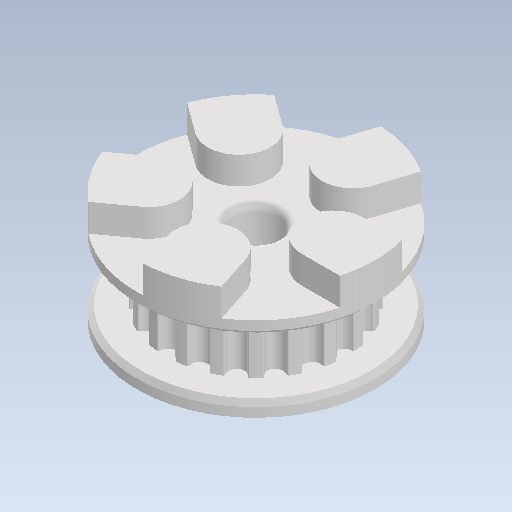
# Autodesk Inventor part: Riemenscheibe HTD_3M
Saved by Autodesk Inventor 2026.4 (Build 304435030, 435C)
## iProperties
Created: 2026-11-19
Part Number: Riemenscheibe HTD_3M
Material: Generisch
Document SubType Name: Modeling
Designer: weira
Density: 1 g/cm^3
Appearance: Vorgabe
Author: weira
Autodesk Inventor part; units mm, degrees
ref_plane "YZ Plane" through (0, 0, 0) normal (1, 0, 0) x (0, 1, 0)
ref_plane "XZ Plane" through (0, 0, 0) normal (0, 1, 0) x (-1, 0, 0)
ref_plane "XY Plane" through (0, 0, 0) normal (0, 0, 1) x (1, 0, 0)
sketch "Skizze1" plane through (0, 0, 0) normal (0, 0, 1) x (1, 0, 0)
  circle A0 centre (0, 0) radius 9.5511 construction
  line L0 (-5.6581, 20.033) -> (2.8903, 20.033)
  line L1 (2.8903, 20.033) -> (2.8903, 11.5277)
  line L2 (2.8903, 11.5277) -> (-5.6581, 11.5277)
  line L3 (-5.6581, 11.5277) -> (-5.6581, 20.033)
  circle A1 centre (0, 0) radius 8.6811 construction
  circle A2 centre (0, 0) radius 9.8211
  arc A3 (0.7095, 9.0476) -> (0.9041, 9.6681) centre (-0.61, 9.8021) ccw
  arc A4 (1.0279, 9.7672) -> (0.9041, 9.6681) centre (1.0264, 9.6422) ccw
  line L4 (0, 8.6811) -> (0, 7.1512) construction
  arc A5 (-0.9041, 9.6681) -> (-0.7095, 9.0476) centre (0.61, 9.8021) ccw
  arc A6 (-0.9041, 9.6681) -> (-1.0279, 9.7672) centre (-1.0264, 9.6422) ccw
  arc A7 (-0.7095, 9.0476) -> (0.7095, 9.0476) centre (0, 9.5511) ccw
  arc A8 (-2.0407, 9.6068) -> (-2.1278, 9.4743) centre (-2.0035, 9.4874) ccw
  arc A9 (-3.8474, 8.9155) -> (-3.9958, 8.9715) centre (-3.9557, 8.8531) ccw
  arc A10 (-2.1211, 8.824) -> (-2.1278, 9.4743) centre (-3.6092, 9.1339) ccw
  arc A11 (-3.8474, 8.9155) -> (-3.4706, 8.3855) centre (-2.4489, 9.5109) ccw
  arc A12 (-3.4706, 8.3855) -> (-2.1211, 8.824) centre (-2.9515, 9.0836) ccw
  arc A13 (-4.9094, 8.506) -> (-4.9513, 8.353) centre (-4.8372, 8.404) ccw
  arc A14 (-6.4142, 7.2902) -> (-6.5726, 7.2976) centre (-6.4979, 7.1974) ccw
  arc A15 (-4.744, 7.7367) -> (-4.9513, 8.353) centre (-6.2551, 7.5715) ccw
  arc A16 (-6.4142, 7.2902) -> (-5.892, 6.9026) centre (-5.2681, 8.2886) ccw
  arc A17 (-5.892, 6.9026) -> (-4.744, 7.7367) centre (-5.614, 7.727) ccw
  arc A18 (-7.2976, 6.5726) -> (-7.2902, 6.4142) centre (-7.1974, 6.4979) ccw
  arc A19 (-8.353, 4.9513) -> (-8.506, 4.9094) centre (-8.404, 4.8372) ccw
  arc A20 (-6.9026, 5.892) -> (-7.2902, 6.4142) centre (-8.2886, 5.2681) ccw
  arc A21 (-8.353, 4.9513) -> (-7.7367, 4.744) centre (-7.5715, 6.2551) ccw
  arc A22 (-7.7367, 4.744) -> (-6.9026, 5.892) centre (-7.727, 5.614) ccw
  arc A23 (-8.9715, 3.9958) -> (-8.9155, 3.8474) centre (-8.8531, 3.9557) ccw
  arc A24 (-9.4743, 2.1278) -> (-9.6068, 2.0407) centre (-9.4874, 2.0035) ccw
  arc A25 (-8.3855, 3.4706) -> (-8.9155, 3.8474) centre (-9.5109, 2.4489) ccw
  arc A26 (-9.4743, 2.1278) -> (-8.824, 2.1211) centre (-9.1339, 3.6092) ccw
  arc A27 (-8.824, 2.1211) -> (-8.3855, 3.4706) centre (-9.0836, 2.9515) ccw
  arc A28 (-9.7672, 1.0279) -> (-9.6681, 0.9041) centre (-9.6422, 1.0264) ccw
  arc A29 (-9.6681, -0.9041) -> (-9.7672, -1.0279) centre (-9.6422, -1.0264) ccw
  arc A30 (-9.0476, 0.7095) -> (-9.6681, 0.9041) centre (-9.8021, -0.61) ccw
  arc A31 (-9.6681, -0.9041) -> (-9.0476, -0.7095) centre (-9.8021, 0.61) ccw
  arc A32 (-9.0476, -0.7095) -> (-9.0476, 0.7095) centre (-9.5511, 0) ccw
  arc A33 (-9.6068, -2.0407) -> (-9.4743, -2.1278) centre (-9.4874, -2.0035) ccw
  arc A34 (-8.9155, -3.8474) -> (-8.9715, -3.9958) centre (-8.8531, -3.9557) ccw
  arc A35 (-8.824, -2.1211) -> (-9.4743, -2.1278) centre (-9.1339, -3.6092) ccw
  arc A36 (-8.9155, -3.8474) -> (-8.3855, -3.4706) centre (-9.5109, -2.4489) ccw
  arc A37 (-8.3855, -3.4706) -> (-8.824, -2.1211) centre (-9.0836, -2.9515) ccw
  arc A38 (-8.506, -4.9094) -> (-8.353, -4.9513) centre (-8.404, -4.8372) ccw
  arc A39 (-7.2902, -6.4142) -> (-7.2976, -6.5726) centre (-7.1974, -6.4979) ccw
  arc A40 (-7.7367, -4.744) -> (-8.353, -4.9513) centre (-7.5715, -6.2551) ccw
  arc A41 (-7.2902, -6.4142) -> (-6.9026, -5.892) centre (-8.2886, -5.2681) ccw
  arc A42 (-6.9026, -5.892) -> (-7.7367, -4.744) centre (-7.727, -5.614) ccw
  arc A43 (-6.5726, -7.2976) -> (-6.4142, -7.2902) centre (-6.4979, -7.1974) ccw
  arc A44 (-4.9513, -8.353) -> (-4.9094, -8.506) centre (-4.8372, -8.404) ccw
  arc A45 (-5.892, -6.9026) -> (-6.4142, -7.2902) centre (-5.2681, -8.2886) ccw
  arc A46 (-4.9513, -8.353) -> (-4.744, -7.7367) centre (-6.2551, -7.5715) ccw
  arc A47 (-4.744, -7.7367) -> (-5.892, -6.9026) centre (-5.614, -7.727) ccw
  arc A48 (-3.9958, -8.9715) -> (-3.8474, -8.9155) centre (-3.9557, -8.8531) ccw
  arc A49 (-2.1278, -9.4743) -> (-2.0407, -9.6068) centre (-2.0035, -9.4874) ccw
  arc A50 (-3.4706, -8.3855) -> (-3.8474, -8.9155) centre (-2.4489, -9.5109) ccw
  arc A51 (-2.1278, -9.4743) -> (-2.1211, -8.824) centre (-3.6092, -9.1339) ccw
  arc A52 (-2.1211, -8.824) -> (-3.4706, -8.3855) centre (-2.9515, -9.0836) ccw
  arc A53 (-1.0279, -9.7672) -> (-0.9041, -9.6681) centre (-1.0264, -9.6422) ccw
  arc A54 (0.9041, -9.6681) -> (1.0279, -9.7672) centre (1.0264, -9.6422) ccw
  arc A55 (-0.7095, -9.0476) -> (-0.9041, -9.6681) centre (0.61, -9.8021) ccw
  arc A56 (0.9041, -9.6681) -> (0.7095, -9.0476) centre (-0.61, -9.8021) ccw
  arc A57 (0.7095, -9.0476) -> (-0.7095, -9.0476) centre (0, -9.5511) ccw
  arc A58 (2.0407, -9.6068) -> (2.1278, -9.4743) centre (2.0035, -9.4874) ccw
  arc A59 (3.8474, -8.9155) -> (3.9958, -8.9715) centre (3.9557, -8.8531) ccw
  arc A60 (2.1211, -8.824) -> (2.1278, -9.4743) centre (3.6092, -9.1339) ccw
  arc A61 (3.8474, -8.9155) -> (3.4706, -8.3855) centre (2.4489, -9.5109) ccw
  arc A62 (3.4706, -8.3855) -> (2.1211, -8.824) centre (2.9515, -9.0836) ccw
  arc A63 (4.9094, -8.506) -> (4.9513, -8.353) centre (4.8372, -8.404) ccw
  arc A64 (6.4142, -7.2902) -> (6.5726, -7.2976) centre (6.4979, -7.1974) ccw
  arc A65 (4.744, -7.7367) -> (4.9513, -8.353) centre (6.2551, -7.5715) ccw
  arc A66 (6.4142, -7.2902) -> (5.892, -6.9026) centre (5.2681, -8.2886) ccw
  arc A67 (5.892, -6.9026) -> (4.744, -7.7367) centre (5.614, -7.727) ccw
  arc A68 (7.2976, -6.5726) -> (7.2902, -6.4142) centre (7.1974, -6.4979) ccw
  arc A69 (8.353, -4.9513) -> (8.506, -4.9094) centre (8.404, -4.8372) ccw
  arc A70 (6.9026, -5.892) -> (7.2902, -6.4142) centre (8.2886, -5.2681) ccw
  arc A71 (8.353, -4.9513) -> (7.7367, -4.744) centre (7.5715, -6.2551) ccw
  arc A72 (7.7367, -4.744) -> (6.9026, -5.892) centre (7.727, -5.614) ccw
  arc A73 (8.9715, -3.9958) -> (8.9155, -3.8474) centre (8.8531, -3.9557) ccw
  arc A74 (9.4743, -2.1278) -> (9.6068, -2.0407) centre (9.4874, -2.0035) ccw
  arc A75 (8.3855, -3.4706) -> (8.9155, -3.8474) centre (9.5109, -2.4489) ccw
  arc A76 (9.4743, -2.1278) -> (8.824, -2.1211) centre (9.1339, -3.6092) ccw
  arc A77 (8.824, -2.1211) -> (8.3855, -3.4706) centre (9.0836, -2.9515) ccw
  arc A78 (9.7672, -1.0279) -> (9.6681, -0.9041) centre (9.6422, -1.0264) ccw
  arc A79 (9.6681, 0.9041) -> (9.7672, 1.0279) centre (9.6422, 1.0264) ccw
  arc A80 (9.0476, -0.7095) -> (9.6681, -0.9041) centre (9.8021, 0.61) ccw
  arc A81 (9.6681, 0.9041) -> (9.0476, 0.7095) centre (9.8021, -0.61) ccw
  arc A82 (9.0476, 0.7095) -> (9.0476, -0.7095) centre (9.5511, 0) ccw
  arc A83 (9.6068, 2.0407) -> (9.4743, 2.1278) centre (9.4874, 2.0035) ccw
  arc A84 (8.9155, 3.8474) -> (8.9715, 3.9958) centre (8.8531, 3.9557) ccw
  arc A85 (8.824, 2.1211) -> (9.4743, 2.1278) centre (9.1339, 3.6092) ccw
  arc A86 (8.9155, 3.8474) -> (8.3855, 3.4706) centre (9.5109, 2.4489) ccw
  arc A87 (8.3855, 3.4706) -> (8.824, 2.1211) centre (9.0836, 2.9515) ccw
  arc A88 (8.506, 4.9094) -> (8.353, 4.9513) centre (8.404, 4.8372) ccw
  arc A89 (7.2902, 6.4142) -> (7.2976, 6.5726) centre (7.1974, 6.4979) ccw
  arc A90 (7.7367, 4.744) -> (8.353, 4.9513) centre (7.5715, 6.2551) ccw
  arc A91 (7.2902, 6.4142) -> (6.9026, 5.892) centre (8.2886, 5.2681) ccw
  arc A92 (6.9026, 5.892) -> (7.7367, 4.744) centre (7.727, 5.614) ccw
  arc A93 (6.5726, 7.2976) -> (6.4142, 7.2902) centre (6.4979, 7.1974) ccw
  arc A94 (4.9513, 8.353) -> (4.9094, 8.506) centre (4.8372, 8.404) ccw
  arc A95 (5.892, 6.9026) -> (6.4142, 7.2902) centre (5.2681, 8.2886) ccw
  arc A96 (4.9513, 8.353) -> (4.744, 7.7367) centre (6.2551, 7.5715) ccw
  arc A97 (4.744, 7.7367) -> (5.892, 6.9026) centre (5.614, 7.727) ccw
  arc A98 (3.9958, 8.9715) -> (3.8474, 8.9155) centre (3.9557, 8.8531) ccw
  arc A99 (2.1278, 9.4743) -> (2.0407, 9.6068) centre (2.0035, 9.4874) ccw
  arc A100 (3.4706, 8.3855) -> (3.8474, 8.9155) centre (2.4489, 9.5109) ccw
  arc A101 (2.1278, 9.4743) -> (2.1211, 8.824) centre (3.6092, 9.1339) ccw
  arc A102 (2.1211, 8.824) -> (3.4706, 8.3855) centre (2.9515, 9.0836) ccw
  circle A103 centre (0, 0) radius 12.0811
  point P0 (-2.6826, 8.2562)
  point P1 (-5.1026, 7.0232)
  point P2 (-7.0232, 5.1026)
  point P3 (-8.2562, 2.6826)
  point P4 (-8.6811, 0)
  point P5 (-8.2562, -2.6826)
  point P6 (-7.0232, -5.1026)
  point P7 (-5.1026, -7.0232)
  point P8 (-2.6826, -8.2562)
  point P9 (0, -8.6811)
  point P10 (2.6826, -8.2562)
  point P11 (5.1026, -7.0232)
  point P12 (7.0232, -5.1026)
  point P13 (8.2562, -2.6826)
  point P14 (8.6811, 0)
  point P15 (8.2562, 2.6826)
  point P16 (7.0232, 5.1026)
  point P17 (5.1026, 7.0232)
  point P18 (2.6826, 8.2562)
  point P19 (-2.0407, 9.6068)
  point P20 (-3.9958, 8.9715)
  point P21 (-4.9094, 8.506)
  point P22 (-6.5726, 7.2976)
  point P23 (-8.506, 4.9094)
  point P24 (-9.6068, -2.0407)
  point P25 (-8.506, -4.9094)
  point P26 (-7.2976, -6.5726)
  point P27 (-2.0407, -9.6068)
  point P28 (2.0407, -9.6068)
  point P29 (4.9094, -8.506)
  point P30 (6.5726, -7.2976)
  point P31 (9.6068, -2.0407)
  point P32 (9.6068, 2.0407)
  dimension "d166" = 19.1022
  dimension "d189" = 1.14
  dimension "d190" = 0.61
  dimension "d194" = 0.25
  dimension "d201" = 360
  dimension "d204" = 3.4
  constraints: 220 point on circle, 101 centre point, 5 coincident, 5 symmetric about line, 2 end point, 2 vertical alignment, 1 vertical, 353 other
  measures "d190" horizontal distance of A3.centre A7.centre
  measures "d194" diameter of A4
extrude "Extrusion1" add sketch "Skizze1" along normal mid plane 6.2 contours A79 A81 A82 A80 A78 A2 A74 A76 A77 A75 A73 A69 A71 A72 A70 A68 A64 A66 A67 A65 A63 A59 A61 A62 A60 A58 A54 A56 A57 A55 A53 A49 A51 A52 A50 A48 A44 A46 A47 A45 A43 A39 A41 A42 A40 A38 A34 A36 A37 A35 A33 A29 A31 A32 A30 A28 A24 A26 A27 A25 A23 A19 A21 A22 A20 A18 A14 A16 A17 A15 A13 A9 A11 A12 A10 A8 A6 A5 A7 A3 A4 A99 A101 A102 A100 A98 A94 A96 A97 A95 A93 A89 A91 A92 A90 A88 A84 A86 A87 A85 A83
sketch "Skizze3" plane through (0, 0, 3.1) normal (0, 0, 1) x (1, 0, 0)
  circle A0 centre (0, 0) radius 12.0811 projected
  circle A1 centre (0, 0) radius 13
  dimension "d220" = 26
  constraints: 1 centre point, 1 coincident
  measures "d220" diameter of A1
extrude "Extrusion4" add sketch "Skizze3" along normal blind 1.5 contours A0 | A1
mirror "Spiegeln1" about plane through (0, 0, 0) normal (0, 0, 1) of "Extrusion4"
chamfer "Fasen1" distance 0.5 angle 45 2 edges at (-13, 0, 3.1) (-13, 0, -3.1)
sketch "Skizze7" plane through (0, 0, 4.6) normal (0, 0, 1) x (1, 0, 0)
  circle A0 centre (0, 0) radius 13 projected
hole "Bohrung1" at (0, 0, 4.6) direction (0, 0, -1) diameter 5 end through all
fillet "Rundung1" radius 0.7 1 edges at (0, 2.5, 4.6)
sketch "Skizze8" plane through (0, 0, 4.6) normal (0, 0, 1) x (1, 0, 0)
  spline S0 degree 3 poles (-4.5905, -2.3496) (-4.7239, -2.2359) (-4.8638, -2.1344) (-5.0099, -2.0442) (-5.0258, -2.0343) (-5.0418, -2.0247) (-5.0579, -2.0151) (-5.15, -1.9603) (-5.245, -1.9097) (-5.3419, -1.8639) (-5.4184, -1.8277) (-5.4959, -1.7945) (-5.5741, -1.7644) (-5.7519, -1.696) (-5.9329, -1.6434) (-6.1169, -1.6059) (-6.3011, -1.5683) (-6.49, -1.5459) (-6.6786, -1.5394) (-7.0559, -1.5264) (-7.4282, -1.5754) (-7.7895, -1.6859) (-8.0137, -1.7544) (-8.2277, -1.8449) (-8.4317, -1.9568) (-8.5563, -2.0253) (-8.6773, -2.1018) (-8.7942, -2.1867) knots 0 0 0 0 0.111776 0.111776 0.111776 0.123964 0.123964 0.123964 0.193761 0.193761 0.193761 0.24879 0.24879 0.24879 0.373901 0.373901 0.373901 0.499098 0.499098 0.499098 0.749579 0.749579 0.749579 0.904998 0.904998 0.904998 1 1 1 1
  arc A0 (-3.6531, -3.6397) -> (-4.5905, -2.3496) centre (-6.7957, -4.9374) ccw
  spline S1 degree 3 poles (-4.7973, -7.6881) (-4.6065, -7.5494) (-4.4337, -7.3939) (-4.2781, -7.2224) (-4.1827, -7.1173) (-4.0938, -7.0062) (-4.0115, -6.8888) (-3.7951, -6.5801) (-3.6334, -6.2419) (-3.529, -5.8799) (-3.4768, -5.699) (-3.4395, -5.5127) (-3.418, -5.3262) (-3.3966, -5.1398) (-3.3905, -4.9516) (-3.4003, -4.7616) (-3.4058, -4.6552) (-3.4164, -4.5482) (-3.4321, -4.4418) (-3.4444, -4.3581) (-3.4599, -4.2747) (-3.4784, -4.1923) (-3.5163, -4.0233) (-3.5672, -3.8568) (-3.6317, -3.6928) (-3.6387, -3.6751) (-3.6458, -3.6574) (-3.6531, -3.6397) knots 0 0 0 0 0.154998 0.154998 0.154998 0.25 0.25 0.25 0.5 0.5 0.5 0.625 0.625 0.625 0.75 0.75 0.75 0.819971 0.819971 0.819971 0.875 0.875 0.875 0.987812 0.987812 0.987812 1 1 1 1
  spline S2 degree 3 poles (-6.7957, 1.5374) (-6.7293, 1.5374) (-6.6626, 1.5393) (-6.5293, 1.5472) (-6.4626, 1.5531) (-6.3321, 1.5685) (-6.2683, 1.5779) (-6.1243, 1.6033) (-6.0443, 1.6205) (-5.8859, 1.6604) (-5.8075, 1.6832) (-5.6973, 1.7195) (-5.665, 1.7307) (-5.57, 1.7653) (-5.5074, 1.7902) (-5.3835, 1.8438) (-5.3222, 1.8726) (-5.2026, 1.933) (-5.1442, 1.9647) (-5.0174, 2.0385) (-4.9492, 2.0814) (-4.8165, 2.1717) (-4.7519, 2.2191) (-4.6555, 2.2952) (-4.6228, 2.322) (-4.5905, 2.3496) knots 0 0 0 0 0.084288 0.084288 0.168552 0.168552 0.25 0.25 0.353842 0.353842 0.457054 0.457054 0.5 0.5 0.583967 0.583967 0.667773 0.667773 0.75 0.75 0.849787 0.849787 0.948403 0.948403 1 1 1 1
  spline S3 degree 3 poles (-3.6531, 3.6397) (-3.5862, 3.8017) (-3.5329, 3.9662) (-3.4923, 4.133) (-3.4878, 4.1512) (-3.4836, 4.1694) (-3.4794, 4.1876) (-3.4558, 4.2921) (-3.4371, 4.3982) (-3.4234, 4.5045) (-3.4127, 4.5884) (-3.4051, 4.6724) (-3.4006, 4.7561) (-3.3904, 4.9463) (-3.3963, 5.1347) (-3.4175, 5.3213) (-3.4387, 5.5081) (-3.4758, 5.6947) (-3.5279, 5.876) (-3.6321, 6.2389) (-3.7938, 6.5778) (-4.0104, 6.8873) (-4.1449, 7.0793) (-4.2971, 7.2549) (-4.4666, 7.4143) (-4.5702, 7.5117) (-4.6803, 7.6031) (-4.7973, 7.6881) knots 0 0 0 0 0.111776 0.111776 0.111776 0.123964 0.123964 0.123964 0.193761 0.193761 0.193761 0.24879 0.24879 0.24879 0.373901 0.373901 0.373901 0.499098 0.499098 0.499098 0.749579 0.749579 0.749579 0.904998 0.904998 0.904998 1 1 1 1
  spline S4 degree 3 poles (0.8161, -5.0919) (0.6667, -5.1836) (0.5269, -5.2853) (0.396, -5.3964) (0.3817, -5.4085) (0.3676, -5.4207) (0.3535, -5.433) (0.273, -5.5037) (0.1955, -5.5784) (0.1219, -5.6565) (0.0639, -5.718) (0.0084, -5.7815) (-0.0444, -5.8466) (-0.1645, -5.9945) (-0.2704, -6.1503) (-0.363, -6.3138) (-0.4556, -6.4773) (-0.5353, -6.6501) (-0.5997, -6.8274) (-0.7287, -7.1823) (-0.7971, -7.5515) (-0.8037, -7.9292) (-0.8078, -8.1636) (-0.7879, -8.3951) (-0.7445, -8.6237) (-0.7179, -8.7634) (-0.6825, -8.9021) (-0.6378, -9.0395) knots 0 0 0 0 0.111776 0.111776 0.111776 0.123964 0.123964 0.123964 0.193761 0.193761 0.193761 0.24879 0.24879 0.24879 0.373901 0.373901 0.373901 0.499098 0.499098 0.499098 0.749579 0.749579 0.749579 0.904998 0.904998 0.904998 1 1 1 1
  arc A1 (2.3327, -4.5991) -> (0.8161, -5.0919) centre (2.5957, -7.9889) ccw
  spline S5 degree 3 poles (5.8293, -6.9382) (5.7565, -6.7139) (5.6619, -6.5015) (5.5469, -6.3005) (5.4765, -6.1773) (5.3982, -6.0584) (5.312, -5.944) (5.0853, -5.6427) (4.8136, -5.3845) (4.5016, -5.1733) (4.3456, -5.0677) (4.18, -4.9747) (4.0093, -4.8966) (3.8386, -4.8186) (3.6616, -4.7547) (3.4778, -4.7053) (3.3749, -4.6777) (3.2699, -4.6546) (3.1638, -4.6367) (3.0804, -4.6225) (2.9963, -4.6115) (2.9122, -4.6036) (2.7398, -4.5875) (2.5658, -4.5844) (2.3898, -4.5951) (2.3708, -4.5963) (2.3518, -4.5976) (2.3327, -4.5991) knots 0 0 0 0 0.154998 0.154998 0.154998 0.25 0.25 0.25 0.5 0.5 0.5 0.625 0.625 0.625 0.75 0.75 0.75 0.819971 0.819971 0.819971 0.875 0.875 0.875 0.987812 0.987812 0.987812 1 1 1 1
  spline S6 degree 3 poles (2.5957, 4.5889) (2.7782, 4.5889) (2.9587, 4.6034) (3.3164, 4.6612) (3.4929, 4.7045) (3.8312, 4.8162) (3.9945, 4.8848) (4.3099, 5.0472) (4.4629, 5.1419) (4.7483, 5.3511) (4.8816, 5.4658) (5.13, 5.7154) (5.2458, 5.8514) (5.558, 6.2827) (5.7184, 6.5969) (5.8293, 6.9382) knots 0 0 0 0 0.125 0.125 0.25 0.25 0.375 0.375 0.5 0.5 0.625 0.625 0.75 0.75 1 1 1 1
  arc A2 (0.8161, 5.0919) -> (2.3327, 4.5991) centre (2.5957, 7.9889) ccw
  spline S7 degree 3 poles (-0.6378, 9.0395) (-0.7107, 8.8152) (-0.7591, 8.5879) (-0.7842, 8.3576) (-0.7996, 8.2166) (-0.8062, 8.0744) (-0.8038, 7.9311) (-0.7974, 7.5541) (-0.7294, 7.1855) (-0.6011, 6.8313) (-0.537, 6.6542) (-0.4576, 6.4815) (-0.3654, 6.3181) (-0.2732, 6.1546) (-0.1676, 5.9988) (-0.0479, 5.8509) (0.0191, 5.768) (0.0905, 5.6877) (0.1658, 5.6108) (0.225, 5.5503) (0.2865, 5.492) (0.3499, 5.4362) (0.4799, 5.3218) (0.6189, 5.217) (0.7675, 5.1222) (0.7836, 5.112) (0.7998, 5.1019) (0.8161, 5.0919) knots 0 0 0 0 0.154998 0.154998 0.154998 0.25 0.25 0.25 0.5 0.5 0.5 0.625 0.625 0.625 0.75 0.75 0.75 0.819971 0.819971 0.819971 0.875 0.875 0.875 0.987812 0.987812 0.987812 1 1 1 1
  spline S8 degree 3 poles (8.4, 3.4) (8.0196, 3.4) (7.6511, 3.3379) (7.2939, 3.2151) (7.2933, 3.2149) (6.9368, 3.0921) (6.6079, 2.9138) (6.3101, 2.6818) (6.309, 2.681) (6.1605, 2.5651) (6.022, 2.4372) (5.8948, 2.2987) (5.8937, 2.2975) (5.767, 2.1591) (5.6525, 2.0117) (5.5487, 1.852) (5.5477, 1.8505) (5.4897, 1.7611) (5.4365, 1.6698) (5.3482, 1.5012) (5.3117, 1.4247) (5.2776, 1.3456) (5.277, 1.3442) (5.2056, 1.1782) (5.1476, 1.0076) (5.1002, 0.8196) (5.0975, 0.8085) (5.0948, 0.7974) knots 0 0 0 0 0.25 0.25 0.250421 0.250421 0.5 0.5 0.500902 0.500902 0.625 0.625 0.626099 0.626099 0.75 0.75 0.75121 0.75121 0.819971 0.819971 0.875 0.875 0.876036 0.876036 0.992705 0.992705 1 1 1 1
  arc A3 (5.0948, 0.7974) -> (5.0948, -0.7974) centre (8.4, 0) ccw
  spline S9 degree 3 poles (5.0948, -0.7974) (5.1377, -0.9752) (5.1941, -1.1465) (5.2676, -1.3221) (5.2719, -1.3324) (5.277, -1.3442) (5.2776, -1.3456) (5.3201, -1.444) (5.3666, -1.5393) (5.4579, -1.7061) (5.5011, -1.7786) (5.5477, -1.8505) (5.5487, -1.852) (5.6525, -2.0117) (5.767, -2.1591) (5.8937, -2.2975) (5.8948, -2.2987) (6.022, -2.4372) (6.1605, -2.5651) (6.309, -2.681) (6.3101, -2.6818) (6.6079, -2.9138) (6.9368, -3.0921) (7.2933, -3.2149) (7.2939, -3.2151) (7.6511, -3.3379) (8.0196, -3.4) (8.4, -3.4) knots 0 0 0 0 0.116669 0.116669 0.123964 0.123964 0.125 0.125 0.193761 0.193761 0.24879 0.24879 0.25 0.25 0.373901 0.373901 0.375 0.375 0.499098 0.499098 0.5 0.5 0.749579 0.749579 0.75 0.75 1 1 1 1
  arc A4 (-4.5905, 2.3496) -> (-3.6531, 3.6397) centre (-6.7957, 4.9374) ccw
  ellipse E0 centre (2.4116, 7.522) end of major axis (5.4117, 6.4598) minor radius 2.9004 (2.3327, 4.5991) -> (2.5957, 4.5889) ccw
  spline S10 degree 3 poles (-8.7942, 2.1867) (-8.5019, 1.9744) (-8.1852, 1.8138) (-7.6754, 1.6483) (-7.5006, 1.6065) (-7.1505, 1.5513) (-6.9739, 1.5374) (-6.7957, 1.5374) knots 0 0 0 0 0.5 0.5 0.75 0.75 1 1 1 1
  circle A5 centre (0, 0) radius 2.3
  circle A6 centre (2.5957, 7.9889) radius 3.4
  circle A7 centre (-6.7957, 4.9374) radius 3.4
  circle A8 centre (-6.7957, -4.9374) radius 3.4
  circle A9 centre (2.5957, -7.9889) radius 3.4
  circle A10 centre (8.4, 0) radius 3.4
  circle A11 centre (-6.7957, 4.9374) radius 3.4
  line L0 (0, 0) -> (2.5957, 7.9889)
  line L1 (2.5957, 7.9889) -> (5.3509, 16.4683) construction
  line L2 (5.8294, 6.9382) -> (8.5845, 15.4177)
  line L3 (2.1173, 17.519) -> (-0.6379, 9.0395)
  arc A12 (-0.6379, 9.0395) -> (5.8294, 6.9382) centre (2.5957, 7.9889) ccw
  arc A13 (8.5845, 15.4177) -> (2.1173, 17.519) centre (5.3509, 16.4683) ccw
  circle A14 centre (0, 0) radius 13
  circle A15 centre (0, 0) radius 3.2
  circle A16 centre (0, 0) radius 13
  point P0 (27.5488, 15.3955)
  point P1 (-0.0203, -2.2999)
  point P2 (-0.4051, -6.3904)
  point P3 (-0.5692, -6.7468)
  point P4 (4.4219, -5.1209)
  point P5 (4.0952, -4.9374)
  point P6 (-6.7334, -1.538)
  point P7 (-3.5337, -5.896)
  point P8 (-3.415, -5.2989)
  point P9 (-3.6531, -3.6397)
  point P10 (-5.6349, -1.7417)
  point P11 (5.0948, -0.7974)
  point P12 (5.2732, -1.3353)
  point P13 (5.5454, -1.847)
  point P14 (5.8982, -2.3024)
  point P15 (6.2991, -2.6732)
  point P16 (6.3013, 2.6749)
  point P17 (5.896, 2.3)
  point P18 (5.5495, 1.8533)
  point P19 (5.0976, 0.8087)
  point P20 (5.0948, 0.7974)
  point P21 (5.4245, 6.1025)
  point P22 (-0.7456, 8.6181)
  point P23 (-0.7978, 7.7792)
  point P24 (-0.6497, 6.9754)
  point P25 (3.9733, 12.2286)
  point P26 (7.111, 10.8827)
  point P27 (0.6438, 12.9841)
  constraints: 14 point on circle, 13 centre point, 10 end point, 6 coincident, 4 tangent, 1 midpoint, 1 parallel, 28 other
extrude "Extrusion7" add sketch "Skizze8" along normal blind 3 contours E0 A2 S7 A6 S6 | A6 L3 A14 L2
pattern_circular "Runde Anordnung1" count 5 over 360 about axis through (0, 0, -33.303) along (0, 0, 1) of "Extrusion7"
